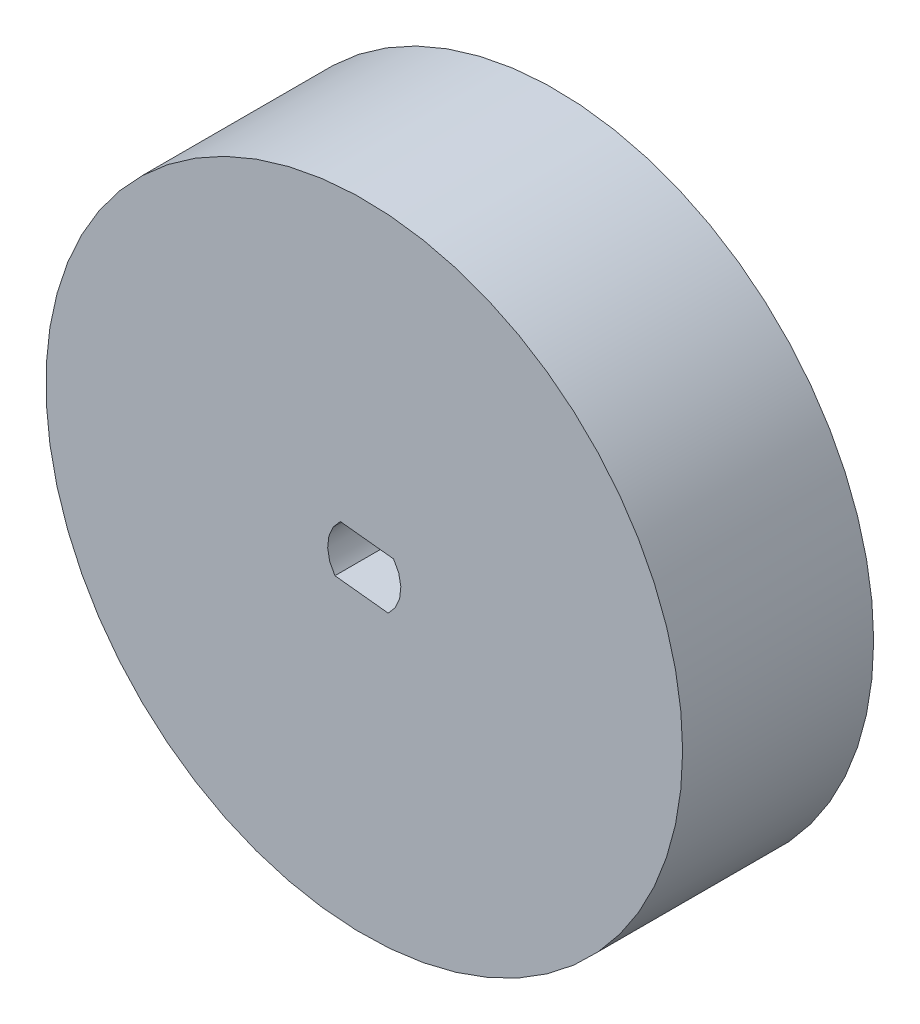
# Autodesk Inventor part: Wheel
Saved by Autodesk Inventor 2024 (Build 280153000, 153)
## iProperties
Created: 2025-06-20
Part Number: Wheel
Material: Generic
Document SubType Name: Modeling
Designer: Aidan
Density: 1 g/cm^3
Appearance: Default
Author: Aidan
Autodesk Inventor part; units mm, degrees
ref_plane "YZ Plane" through (0, 0, 0) normal (1, 0, 0) x (0, 1, 0)
ref_plane "XZ Plane" through (0, 0, 0) normal (0, 1, 0) x (-1, 0, 0)
ref_plane "XY Plane" through (0, 0, 0) normal (0, 0, 1) x (1, 0, 0)
sketch "Sketch1" plane through (0, 0, 0) normal (0, 0, 1) x (1, 0, 0)
  arc A0 (3.5672, 9.7088) -> (3.9466, 13.2083) centre (1.7542, 11.6757) ccw projected
  line L0 (3.9466, 13.2083) -> (-0.0588, 13.6426) projected
  arc A1 (-0.0588, 13.6426) -> (-0.4383, 10.1432) centre (1.7542, 11.6757) ccw projected
  line L1 (-0.4383, 10.1432) -> (3.5672, 9.7088) projected
  circle A2 centre (1.7542, 11.6757) radius 1.04 projected
  circle A3 centre (1.7542, 11.6757) radius 25
  line L2 (-0.1256, 13.8511) -> (4.0565, 13.3976)
  arc A4 (3.634, 9.5004) -> (4.0565, 13.3976) centre (1.7542, 11.6757) ccw
  line L3 (3.634, 9.5004) -> (-0.5482, 9.9539)
  arc A5 (-0.1256, 13.8511) -> (-0.5482, 9.9539) centre (1.7542, 11.6757) ccw
  point P0 (0, 0)
  dimension "d0" = 50
  dimension "d1" = 0.2
  constraints: 4 end point, 4 point on circle, 3 centre point, 1 coincident, 3 other
  measures "d0" diameter of A3
  measures "d1" distance between parallel lines of L0 L2
extrude "Extrusion1" add sketch "Sketch1" along normal blind 15 contours A3
body "Solid1"
